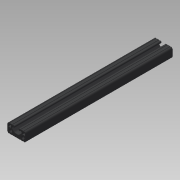
# Autodesk Inventor part: 1534-LITE
Saved by Autodesk Inventor 2013 (Build 170138000, 138)
## iProperties
Company: 80/20 Inc.
Created: 2014-04-23
Part Number: 1534-LITE
Material: Generic
Document SubType Name: Modeling
Density: 1 g/cm^3
Vendor: 80/20 Inc.
Engineer: Ross Bowman
Designer: Ross Bowman
Catalog Web Link: 8020.net
Material: 6105-T5 Aluminum
Author: Ross Bowman
Keywords: 80/20 , 8020 , T-Slot , Extrusion
Autodesk Inventor part; units mm, degrees
ref_plane "YZ Plane" through (0, 0, 0) normal (1, 0, 0) x (0, 1, 0)
ref_plane "XZ Plane" through (0, 0, 0) normal (0, 1, 0) x (-1, 0, 0)
ref_plane "XY Plane" through (0, 0, 0) normal (0, 0, 1) x (1, 0, 0)
sketch "Sketch1" plane through (0, 0, 0) normal (0, 0, 1) x (1, 0, 0)
  circle A0 centre (12.7, -3.175) radius 3.3274
  arc A1 (-12.1461, 2.3151) -> (-11.8921, 2.5691) centre (-12.1461, 2.5691) ccw
  line L0 (-17.0229, 2.3151) -> (-12.1461, 2.3151)
  arc A2 (-17.2769, 2.5691) -> (-17.0229, 2.3151) centre (-17.0229, 2.5691) ccw
  line L1 (-17.2769, 4.9059) -> (-17.2769, 2.5691)
  arc A3 (-14.4829, 7.6999) -> (-17.2769, 4.9059) centre (-14.4829, 4.9059) ccw
  line L2 (-12.1461, 7.6999) -> (-14.4829, 7.6999)
  arc A4 (-11.8921, 7.4459) -> (-12.1461, 7.6999) centre (-12.1461, 7.4459) ccw
  line L3 (-11.8921, 2.5691) -> (-11.8921, 7.4459)
  circle A5 centre (-12.7, -3.175) radius 3.3274
  arc A6 (12.1461, 7.6999) -> (11.8921, 7.4459) centre (12.1461, 7.4459) ccw
  line L4 (14.4829, 7.6999) -> (12.1461, 7.6999)
  arc A7 (17.2769, 4.9059) -> (14.4829, 7.6999) centre (14.4829, 4.9059) ccw
  line L5 (17.2769, 2.5691) -> (17.2769, 4.9059)
  arc A8 (17.0229, 2.3151) -> (17.2769, 2.5691) centre (17.0229, 2.5691) ccw
  line L6 (12.1461, 2.3151) -> (17.0229, 2.3151)
  arc A9 (11.8921, 2.5691) -> (12.1461, 2.3151) centre (12.1461, 2.5691) ccw
  line L7 (11.8921, 7.4459) -> (11.8921, 2.5691)
  line L8 (-9.4427, 9.525) -> (-14.0829, 9.525)
  arc A10 (-15.6028, 9.525) -> (-14.0829, 9.525) centre (-14.8428, 9.525) ccw
  line L9 (-15.6028, 9.525) -> (-15.875, 9.525)
  arc A11 (-15.875, 9.525) -> (-19.05, 6.35) centre (-15.875, 6.35) ccw
  line L10 (-19.05, 6.35) -> (-19.05, -6.35)
  arc A12 (-19.05, -6.35) -> (-15.875, -9.525) centre (-15.875, -6.35) ccw
  line L11 (-15.875, -9.525) -> (-15.6028, -9.525)
  arc A13 (-14.0829, -9.525) -> (-15.6028, -9.525) centre (-14.8428, -9.525) ccw
  line L12 (-14.0829, -9.525) -> (-9.4578, -9.525)
  arc A14 (-7.9379, -9.525) -> (-9.4578, -9.525) centre (-8.6979, -9.525) ccw
  line L13 (-7.9379, -9.525) -> (7.9379, -9.525)
  arc A15 (9.4578, -9.525) -> (7.9379, -9.525) centre (8.6979, -9.525) ccw
  line L14 (9.4578, -9.525) -> (14.0829, -9.525)
  arc A16 (15.6028, -9.525) -> (14.0829, -9.525) centre (14.8428, -9.525) ccw
  line L15 (15.6028, -9.525) -> (15.875, -9.525)
  arc A17 (15.875, -9.525) -> (19.05, -6.35) centre (15.875, -6.35) ccw
  line L16 (19.05, -6.35) -> (19.05, 6.35)
  arc A18 (19.05, 6.35) -> (15.875, 9.525) centre (15.875, 6.35) ccw
  line L17 (15.875, 9.525) -> (15.6028, 9.525)
  arc A19 (14.0829, 9.525) -> (15.6028, 9.525) centre (14.8428, 9.525) ccw
  line L18 (14.0829, 9.525) -> (9.4427, 9.525)
  arc A20 (7.9228, 9.525) -> (9.4427, 9.525) centre (8.6828, 9.525) ccw
  line L19 (7.9228, 9.525) -> (5.6388, 9.525)
  arc A21 (5.6388, 9.525) -> (4.064, 7.9502) centre (5.6388, 7.9502) ccw
  line L20 (4.064, 7.9502) -> (4.064, 7.0358)
  arc A22 (4.064, 7.0358) -> (5.6388, 5.461) centre (5.6388, 7.0358) ccw
  line L21 (5.6388, 5.461) -> (6.6706, 5.461)
  arc A23 (6.6706, 5.461) -> (6.9246, 5.715) centre (6.6706, 5.715) ccw
  line L22 (6.9246, 5.715) -> (6.9246, 6.081)
  arc A24 (7.1786, 6.335) -> (6.9246, 6.081) centre (7.1786, 6.081) ccw
  line L23 (7.1786, 6.335) -> (9.017, 6.335)
  arc A25 (10.287, 5.065) -> (9.017, 6.335) centre (9.017, 5.065) ccw
  line L24 (10.287, 5.065) -> (10.287, 3.6128)
  arc A26 (10.0266, 2.9842) -> (10.287, 3.6128) centre (9.398, 3.6128) ccw
  line L25 (10.0266, 2.9842) -> (5.6159, -1.4264)
  arc A27 (2.621, -2.667) -> (5.6159, -1.4264) centre (2.621, 1.5686) ccw
  line L26 (2.621, -2.667) -> (-2.621, -2.667)
  arc A28 (-5.6159, -1.4264) -> (-2.621, -2.667) centre (-2.621, 1.5686) ccw
  line L27 (-5.6159, -1.4264) -> (-10.0266, 2.9842)
  arc A29 (-10.287, 3.6128) -> (-10.0266, 2.9842) centre (-9.398, 3.6128) ccw
  line L28 (-10.287, 3.6128) -> (-10.287, 5.065)
  arc A30 (-9.017, 6.335) -> (-10.287, 5.065) centre (-9.017, 5.065) ccw
  line L29 (-9.017, 6.335) -> (-7.1786, 6.335)
  arc A31 (-6.9246, 6.081) -> (-7.1786, 6.335) centre (-7.1786, 6.081) ccw
  line L30 (-6.9246, 6.081) -> (-6.9246, 5.715)
  arc A32 (-6.9246, 5.715) -> (-6.6706, 5.461) centre (-6.6706, 5.715) ccw
  line L31 (-6.6706, 5.461) -> (-5.6388, 5.461)
  arc A33 (-5.6388, 5.461) -> (-4.064, 7.0358) centre (-5.6388, 7.0358) ccw
  line L32 (-4.064, 7.0358) -> (-4.064, 7.9502)
  arc A34 (-4.064, 7.9502) -> (-5.6388, 9.525) centre (-5.6388, 7.9502) ccw
  line L33 (-5.6388, 9.525) -> (-7.9228, 9.525)
  arc A35 (-9.4427, 9.525) -> (-7.9228, 9.525) centre (-8.6828, 9.525) ccw
  point P0 (0, 0)
  constraints: 68 end point, 68 point on circle, 36 centre point
extrude "Extrusion1" add sketch "Sketch1" against normal blind 304.8
body "Solid1"
